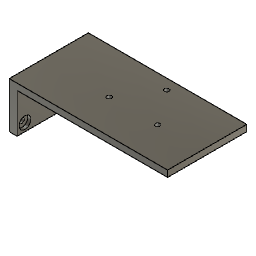
Boat_final_design v3 (Autodesk Fusion 360 archive; units mm, degrees)
design "Plat_servo_cover"
Autodesk Fusion 360 part; units mm, degrees
(part 1 of 7)
sketch "Sketch1" plane through (0, 0, 0) normal (0, 0, 1) x (1, 0, 0)
  line L0 (50, 25) -> (-50, 25)
  line L1 (-50, 25) -> (-50, -25)
  line L2 (-50, -25) -> (50, -25)
  line L3 (50, -25) -> (50, 25)
  line L4 (50, 25) -> (-50, -25) construction
  line L5 (-50, 25) -> (50, -25) construction
  line L6 (-50, 25) -> (-45, 25)
  line L7 (-45, 25) -> (-45, -24.9653)
  line L8 (-45, -24.9653) -> (-50, -24.9653)
  line L9 (-50, -24.9653) -> (-50, 25)
  dimension "d1" = 100
  dimension "d2" = 50
  dimension "d5" = 5
  constraint horizontal L0
  constraint perpendicular L0 L1
  constraint parallel L0 L2
  constraint parallel L1 L3
  constraint coincident L4 origin
  constraint coincident L5 origin
  constraint horizontal L6
  constraint vertical L7
  constraint horizontal L8
  constraint vertical L9
  measures "d1" distance of L1.end L2.end
  measures "d2" distance of L0.end L1.end
  measures "d5" distance of L0.end L6.end
extrude "Extrude1" add sketch "Sketch1" along normal blind 4 makes body 1
extrude "Extrude2" add sketch "Sketch1" against normal blind 25 contours L0 L1 L6 L7 L8 L9 bodies 1
sketch "Sketch2" plane through (0, 0, 0) normal (0, 0, 1) x (1, 0, 0)
  circle A0 centre (-33.372, 3.4391) radius 6.25
  circle A1 centre (-33.372, 9.4391) radius 3.25
  line L0 (50, 25) -> (-50, 25)
  line L1 (-50, -25) -> (50, -25)
  line L2 (-50, -24.9653) -> (-50, 25)
  line L3 (-45, -7.5609) -> (-27.5, -7.5609)
  line L4 (-27.5, -7.5609) -> (-27.5, -2.7609)
  line L5 (-27.5, -2.7609) -> (-45, -2.7609)
  line L6 (-45, -2.7609) -> (-45, -7.5609)
  circle A2 centre (-13.372, 3.4391) radius 3.25
  circle A3 centre (6.628, 3.4391) radius 3.25
  line L7 (-44.814, 24.8891) -> (-27.314, 24.8891)
  line L8 (-27.314, 24.8891) -> (-27.314, 20.0891)
  line L9 (-27.314, 20.0891) -> (-44.814, 20.0891)
  line L10 (-44.814, 20.0891) -> (-44.814, 24.8891)
  dimension "d8" = 12.5
  dimension "d9" = 6.5
  dimension "d15" = 6
  dimension "d17" = 16.628
  dimension "d20" = 17.5
  dimension "d21" = 4.8
  dimension "d47" = 6.5
  dimension "d48" = 20
  dimension "d49" = 6.5
  dimension "d50" = 20
  dimension "d54" = 11
  dimension "d55" = 17.5
  dimension "d56" = 4.8
  dimension "d57" = 32.45
  constraint vertical A0.centre A1.centre
  constraint horizontal L3
  constraint vertical L4
  constraint horizontal L5
  constraint vertical L6
  constraint horizontal A0.centre A2.centre
  constraint horizontal A2.centre A3.centre
  constraint horizontal L7
  constraint vertical L8
  constraint horizontal L9
  constraint vertical L10
  measures "d8" diameter of A0
  measures "d9" diameter of A1
  measures "d15" distance of A0.centre A1.centre
  measures "d17" distance of A0.centre L2
  measures "d20" distance of L3.start L3.end
  measures "d21" distance of L3.start L5.end
  measures "d47" diameter of A2
  measures "d48" horizontal distance of A0.centre A2.centre
  measures "d49" diameter of A3
  measures "d50" horizontal distance of A2.centre A3.centre
  measures "d54" distance of A0.centre L3
  measures "d55" distance of L7.start L7.end
  measures "d56" distance of L7.start L9.end
  measures "d57" distance of L3 L7
sketch "Sketch5" plane through (-45, 0, 0) normal (1, 0, 0) x (0, 1, 0)
  line L0 (-24.9653, 0) -> (-24.9653, -25)
  line L1 (-24.9653, -25) -> (25, -25)
  line L2 (25, -25) -> (25, 0)
  line L3 (25, 0) -> (-24.9653, 0)
  circle A0 centre (20, -20) radius 1.5
  circle A1 centre (-20, -20) radius 1.5
  circle A2 centre (20, -20) radius 3.75
  circle A3 centre (-20, -20) radius 3.75
  line L4 (-8, -9) -> (25, -9)
  line L5 (25, -9) -> (25, -16)
  line L6 (25, -16) -> (-8, -16)
  line L7 (-8, -16) -> (-8, -9)
  dimension "d37" = 3
  dimension "d38" = 3
  dimension "d39" = 5
  dimension "d40" = 40
  dimension "d43" = 7.5
  dimension "d44" = 7.5
  constraint horizontal A0.centre A1.centre
  constraint concentric A0 A2
  constraint concentric A1 A3
  constraint horizontal L4
  constraint vertical L5
  constraint horizontal L6
  constraint vertical L7
  constraint coincident L2 L4.end
  measures "d37" diameter of A0
  measures "d38" diameter of A1
  measures "d39" distance of L1 A0.centre
  measures "d40" distance of A0.centre A1.centre
  measures "d43" diameter of A2
  measures "d44" diameter of A3
extrude "Extrude7" cut sketch "Sketch5" against normal blind 19 contours A0 | A1 bodies 1
extrude "Extrude8" cut sketch "Sketch5" against normal blind 2 contours A2 | A3 bodies 1
sketch "Sketch6" plane through (0, 0, 4) normal (0, 0, 1) x (-1, 0, 0)
  line L0 (50, -25) -> (50, 25)
  line L1 (50, 25) -> (-50, 25)
  line L2 (-50, 25) -> (-50, -25)
  line L3 (-50, -25) -> (50, -25)
  circle A0 centre (8.372, -3.4391) radius 6
  circle A1 centre (-22.128, -3.4391) radius 6
  circle A2 centre (-22.128, -3.4391) radius 1.5
  line L4 (-50, 12.8409) -> (-13.2169, 12.8409) construction
  line L5 (-50, 16.0661) -> (-11, 16.0661) construction
  line L6 (-13.2169, 12.8409) -> (1.2489, 12.8409)
  line L7 (1.2489, 12.8409) -> (1.2489, 24)
  line L8 (1.2489, 24) -> (-13.2169, 24)
  line L9 (-13.2169, 24) -> (-13.2169, 12.8409)
  line L10 (-5.984, 12.8409) -> (-5.984, 24) construction
  line L11 (1.2489, 18.4205) -> (-13.2169, 18.4205) construction
  circle A3 centre (8.372, -3.4391) radius 1.5
  circle A4 centre (-5.984, 18.4205) radius 1.5
  dimension "d80" = 12
  dimension "d93" = 12
  dimension "d94" = 3
  dimension "d98" = 30.5
  dimension "d129" = 1
  dimension "d131" = 3
  dimension "d193" = 3
  constraint concentric A1 A2
  constraint coincident L2 L4.start
  constraint perpendicular L2 L4
  constraint horizontal L5
  constraint coincident L2 L5.start
  constraint horizontal L6
  constraint vertical L7
  constraint horizontal L8
  constraint vertical L9
  constraint midpoint L6 L10.start
  constraint midpoint L8 L10.end
  constraint midpoint L7 L11.start
  constraint midpoint L9 L11.end
  constraint concentric A0 A3
  constraint horizontal A0.centre A1.centre
  constraint midpoint L10 A4.centre
  measures "d80" diameter of A0
  measures "d93" diameter of A1
  measures "d94" diameter of A2
  measures "d98" distance of A0.centre A1.centre
  measures "d129" distance of L1 L8
  measures "d131" diameter of A3
  measures "d193" diameter of A4
extrude "Extrude23" cut sketch "Sketch6" against normal blind 13 contours A2 | A3 | A4 bodies 1
mirror "Mirror1" about plane through (-50, -25, 0) normal (0, -1, 0) of bodies 1 makes body 2
move_body "Move1" bodies 1 to x (1, 0, 0) y (0, 1, 0) z (0, 0, 1) at (0, 35, 0)
hidden bodies 1

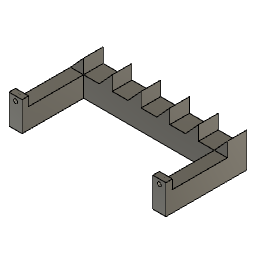
design "Wall_reverse"
Autodesk Fusion 360 part; units mm, degrees
sketch "Sketch1" plane through (0, 0, 0) normal (0, 0, 1) x (1, 0, 0)
  line L0 (30, -7.5) -> (-30, -7.5)
  line L1 (-30, -7.5) -> (-30, 7.5)
  line L2 (-30, 7.5) -> (30, 7.5)
  line L3 (30, 7.5) -> (30, -7.5)
  line L4 (30, -7.5) -> (-30, 7.5) construction
  line L5 (-30, -7.5) -> (30, 7.5) construction
  dimension "d1" = 60
  dimension "d2" = 15
  constraint horizontal L0
  constraint perpendicular L0 L1
  constraint parallel L0 L2
  constraint parallel L1 L3
  constraint coincident L4 origin
  constraint coincident L5 origin
  measures "d1" distance of L1.end L2.end
  measures "d2" distance of L0.end L1.end
extrude "Extrude1" add sketch "Sketch1" along normal blind 15.5 makes body 1
sketch "Sketch2" plane through (0, 0, 15.5) normal (0, 0, 1) x (-1, 0, 0)
  line L0 (-30, -7.5) -> (30, -7.5)
  line L1 (30, -7.5) -> (30, 7.5)
  line L2 (30, 7.5) -> (-30, 7.5)
  line L3 (-30, 7.5) -> (-30, -7.5)
  line L4 (-30, -7.5) -> (-15, -7.5)
  line L5 (-15, -7.5) -> (-15, 12.5)
  line L6 (-15, 12.5) -> (-30, 12.5)
  line L7 (-30, 12.5) -> (-30, -7.5)
  dimension "d5" = 15
  dimension "d6" = 20
  constraint horizontal L4
  constraint vertical L5
  constraint horizontal L6
  constraint vertical L7
  constraint coincident L0.start L3.end
  measures "d5" distance of L0.start L4.end
  measures "d6" distance of L0.start L6.end
sketch "Sketch3" plane through (0, -7.5, 0) normal (0, -1, 0) x (1, 0, 0)
  line L0 (-30, 0) -> (30, 0)
  line L1 (30, 0) -> (30, 15.5)
  line L2 (30, 15.5) -> (-30, 15.5)
  line L3 (-30, 15.5) -> (-30, 0)
  line L4 (20, 15.5) -> (30, 15.5)
  line L5 (30, 15.5) -> (30, 0)
  line L6 (30, 0) -> (20, 0)
  line L7 (20, 0) -> (20, 15.5)
  constraint horizontal L4
  constraint vertical L5
  constraint horizontal L6
  constraint vertical L7
  constraint coincident L0.end L1.start
  constraint coincident L1.end L2.start
extrude "Extrude3" add sketch "Sketch3" along normal blind 47 contours L0 L1 L2 L4 L5 L6 L7 bodies 1
sketch "Sketch4" plane through (0, 0, 15.5) normal (0, 0, 1) x (-1, 0, 0)
  line L0 (-30, 54.5) -> (-30, -7.5)
  line L1 (-20, 7.5) -> (-20, 54.5)
  line L2 (-20, 54.5) -> (-30, 54.5)
  line L3 (-20, 54.5) -> (-61.6412, 54.5)
  line L4 (-61.6412, 54.5) -> (-61.6412, 49.5)
  line L5 (-61.6412, 49.5) -> (-20, 49.5)
  line L6 (-20, 49.5) -> (-20, 54.5)
  line L7 (-30, -7.5) -> (30, -7.5)
  line L8 (30, -7.5) -> (30, 7.5)
  line L9 (30, 7.5) -> (-20, 7.5)
  dimension "d11" = 5
  constraint horizontal L3
  constraint vertical L4
  constraint horizontal L5
  constraint vertical L6
  constraint coincident L1.end L2.start
  measures "d11" distance of L1.end L5.end
extrude "Extrude4" add sketch "Sketch4" along normal blind 7 contours L0 L1 L2 L3 L5 L6 bodies 1
mirror "Mirror1" about plane through (-30, -7.5, 0) normal (-1, 0, 0) of bodies 1 merged
sketch "Sketch5" plane through (0, -49.5, 0) normal (0, 1, 0) x (-1, 0, 0)
  line L0 (80, 15.5) -> (90, 15.5)
  line L1 (90, 15.5) -> (90, 22.5)
  line L2 (90, 22.5) -> (80, 22.5)
  line L3 (80, 22.5) -> (80, 15.5)
  circle A0 centre (-25, 19) radius 3
  circle A1 centre (-25, 19) radius 1.5
  circle A2 centre (85, 19) radius 3
  circle A3 centre (85, 19) radius 1.5
  line L4 (-20, 22.5) -> (-30, 22.5)
  line L5 (-20, 15.5) -> (-20, 22.5)
  dimension "d16" = 6
  dimension "d17" = 3
  dimension "d18" = 6
  dimension "d19" = 3
  dimension "d24" = 3.5
  dimension "d25" = 3.5
  dimension "d40" = 5
  dimension "d41" = 5
  constraint concentric A0 A1
  constraint concentric A2 A3
  measures "d16" diameter of A0
  measures "d17" diameter of A1
  measures "d18" diameter of A2
  measures "d19" diameter of A3
  measures "d24" distance of A0.centre L4
  measures "d25" distance of L2 A2.centre
  measures "d40" distance of A0.centre L5
  measures "d41" distance of L1 A2.centre
extrude "Extrude5" cut sketch "Sketch5" against normal blind 15 contours A1 | A3 bodies 1
extrude "Extrude6" cut sketch "Sketch5" against normal blind 2 contours A0 | A2 bodies 1
sketch "Sketch6" plane through (0, 0, 15.5) normal (0, 0, 1) x (-1, 0, 0)
  line L0 (-20, 49.5) -> (-30, 49.5)
  line L1 (-30, 49.5) -> (-30, -7.5)
  line L2 (-30, -7.5) -> (90, -7.5)
  line L3 (90, -7.5) -> (90, 49.5)
  line L4 (90, 49.5) -> (80, 49.5)
  line L5 (80, 49.5) -> (80, 7.5)
  line L6 (80, 7.5) -> (-20, 7.5)
  line L7 (-20, 7.5) -> (-20, 49.5)
  line L8 (-30, -7.5) -> (-20, -7.5)
  line L9 (-20, -7.5) -> (-20, 7.5)
  line L10 (-20, 7.5) -> (-30, 7.5)
  line L11 (-30, 7.5) -> (-30, -7.5)
  constraint horizontal L8
  constraint vertical L9
  constraint horizontal L10
  constraint vertical L11
  constraint coincident L1.end L2.start
  constraint coincident L6.end L7.start
extrude "Extrude7" add sketch "Sketch6" along normal blind 11 contours L1 L2 L8 L9 L10 L11 bodies 1
sketch "Sketch7" plane through (0, -7.5, 0) normal (0, -1, 0) x (1, 0, 0)
  line L0 (20, 15.5) -> (30, 15.5)
  line L1 (30, 15.5) -> (30, 26.5)
  line L2 (30, 26.5) -> (20, 26.5)
  line L3 (20, 26.5) -> (20, 15.5)
  line L4 (20, 26.5) -> (30, 15.5)
  constraint coincident L2.end L3.start
  constraint coincident L0.end L1.start
extrude "Extrude9" cut sketch "Sketch7" against normal through all contours L1 L2 L4 bodies 1
pattern_linear "R-Pattern2" count 6 spacing 22 along (-1, 0, 0) of "Extrude7", "Extrude9"
mirror "Mirror2" about plane through (0, 0, 0) normal (1, 0, 0) of bodies 1 makes body 2
move_body "Move1" bodies 2 to x (1, 0, 0) y (0, 1, 0) z (0, 0, 1) at (-55, 95, 0)
hidden bodies 1

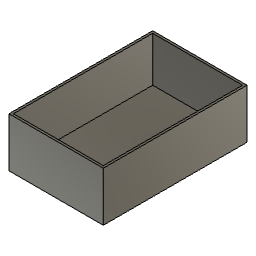
design "ikea box hull"
Autodesk Fusion 360 part; units mm, degrees
sketch "Sketch1" plane through (0, 0, 0) normal (0, 0, 1) x (1, 0, 0)
  line L0 (105, 160) -> (-105, 160)
  line L1 (-105, 160) -> (-105, -160)
  line L2 (-105, -160) -> (105, -160)
  line L3 (105, -160) -> (105, 160)
  line L4 (105, 160) -> (-105, -160) construction
  line L5 (-105, 160) -> (105, -160) construction
  dimension "d1" = 210
  dimension "d2" = 320
  constraint horizontal L0
  constraint perpendicular L0 L1
  constraint parallel L0 L2
  constraint parallel L1 L3
  constraint coincident L4 origin
  constraint coincident L5 origin
  measures "d1" distance of L1.end L2.end
  measures "d2" distance of L0.end L1.end
extrude "Extrude1" add sketch "Sketch1" along normal blind 110
sketch "Sketch2" plane through (0, 0, 110) normal (0, 0, 1) x (-1, 0, 0)
  line L0 (-105, 160) -> (-105, -160)
  line L1 (-105, -160) -> (105, -160)
  line L2 (105, -160) -> (105, 160)
  line L3 (105, 160) -> (-105, 160)
  line L4 (-100, -155) -> (100, -155)
  line L5 (100, -155) -> (100, 155)
  line L6 (100, 155) -> (-100, 155)
  line L7 (-100, 155) -> (-100, -155)
  line L8 (-100, -155) -> (100, 155) construction
  line L9 (100, -155) -> (-100, 155) construction
  dimension "d5" = 200
  dimension "d6" = 310
  constraint horizontal L4
  constraint perpendicular L4 L5
  constraint parallel L4 L6
  constraint parallel L5 L7
  constraint coincident L8 origin
  constraint coincident L9 origin
  measures "d5" distance of L5.end L6.end
  measures "d6" distance of L4.end L5.end
extrude "Extrude2" cut sketch "Sketch2" against normal blind 100 contours L4 L5 L6 L7

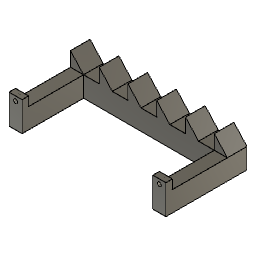
design "Wall"
Autodesk Fusion 360 part; units mm, degrees
sketch "Sketch1" plane through (0, 0, 0) normal (0, 0, 1) x (1, 0, 0)
  line L0 (30, -7.5) -> (-30, -7.5)
  line L1 (-30, -7.5) -> (-30, 7.5)
  line L2 (-30, 7.5) -> (30, 7.5)
  line L3 (30, 7.5) -> (30, -7.5)
  line L4 (30, -7.5) -> (-30, 7.5) construction
  line L5 (-30, -7.5) -> (30, 7.5) construction
  dimension "d1" = 60
  dimension "d2" = 15
  constraint horizontal L0
  constraint perpendicular L0 L1
  constraint parallel L0 L2
  constraint parallel L1 L3
  constraint coincident L4 origin
  constraint coincident L5 origin
  measures "d1" distance of L1.end L2.end
  measures "d2" distance of L0.end L1.end
extrude "Extrude1" add sketch "Sketch1" along normal blind 15.5
sketch "Sketch2" plane through (0, 0, 15.5) normal (0, 0, 1) x (-1, 0, 0)
  line L0 (-30, -7.5) -> (30, -7.5)
  line L1 (30, -7.5) -> (30, 7.5)
  line L2 (30, 7.5) -> (-30, 7.5)
  line L3 (-30, 7.5) -> (-30, -7.5)
  line L4 (-30, -7.5) -> (-15, -7.5)
  line L5 (-15, -7.5) -> (-15, 12.5)
  line L6 (-15, 12.5) -> (-30, 12.5)
  line L7 (-30, 12.5) -> (-30, -7.5)
  dimension "d5" = 15
  dimension "d6" = 20
  constraint horizontal L4
  constraint vertical L5
  constraint horizontal L6
  constraint vertical L7
  constraint coincident L0.start L3.end
  measures "d5" distance of L0.start L4.end
  measures "d6" distance of L0.start L6.end
sketch "Sketch3" plane through (0, -7.5, 0) normal (0, -1, 0) x (1, 0, 0)
  line L0 (-30, 0) -> (30, 0)
  line L1 (30, 0) -> (30, 15.5)
  line L2 (30, 15.5) -> (-30, 15.5)
  line L3 (-30, 15.5) -> (-30, 0)
  line L4 (20, 15.5) -> (30, 15.5)
  line L5 (30, 15.5) -> (30, 0)
  line L6 (30, 0) -> (20, 0)
  line L7 (20, 0) -> (20, 15.5)
  constraint horizontal L4
  constraint vertical L5
  constraint horizontal L6
  constraint vertical L7
  constraint coincident L0.end L1.start
  constraint coincident L1.end L2.start
extrude "Extrude3" add sketch "Sketch3" along normal blind 47 contours L0 L1 L2 L4 L5 L6 L7
sketch "Sketch4" plane through (0, 0, 15.5) normal (0, 0, 1) x (-1, 0, 0)
  line L0 (-30, 54.5) -> (-30, -7.5)
  line L1 (-20, 7.5) -> (-20, 54.5)
  line L2 (-20, 54.5) -> (-30, 54.5)
  line L3 (-20, 54.5) -> (-61.6412, 54.5)
  line L4 (-61.6412, 54.5) -> (-61.6412, 49.5)
  line L5 (-61.6412, 49.5) -> (-20, 49.5)
  line L6 (-20, 49.5) -> (-20, 54.5)
  line L7 (-30, -7.5) -> (30, -7.5)
  line L8 (30, -7.5) -> (30, 7.5)
  line L9 (30, 7.5) -> (-20, 7.5)
  dimension "d11" = 5
  constraint horizontal L3
  constraint vertical L4
  constraint horizontal L5
  constraint vertical L6
  constraint coincident L1.end L2.start
  measures "d11" distance of L1.end L5.end
extrude "Extrude4" add sketch "Sketch4" along normal blind 7 contours L0 L1 L2 L3 L5 L6
mirror "Mirror1" about plane through (-30, -7.5, 0) normal (-1, 0, 0) of bodies 1 merged
sketch "Sketch5" plane through (0, -49.5, 0) normal (0, 1, 0) x (-1, 0, 0)
  line L0 (80, 15.5) -> (90, 15.5)
  line L1 (90, 15.5) -> (90, 22.5)
  line L2 (90, 22.5) -> (80, 22.5)
  line L3 (80, 22.5) -> (80, 15.5)
  circle A0 centre (-25, 19) radius 3
  circle A1 centre (-25, 19) radius 1.5
  circle A2 centre (85, 19) radius 3
  circle A3 centre (85, 19) radius 1.5
  line L4 (-20, 22.5) -> (-30, 22.5)
  line L5 (-20, 15.5) -> (-20, 22.5)
  dimension "d16" = 6
  dimension "d17" = 3
  dimension "d18" = 6
  dimension "d19" = 3
  dimension "d24" = 3.5
  dimension "d25" = 3.5
  dimension "d40" = 5
  dimension "d41" = 5
  constraint concentric A0 A1
  constraint concentric A2 A3
  measures "d16" diameter of A0
  measures "d17" diameter of A1
  measures "d18" diameter of A2
  measures "d19" diameter of A3
  measures "d24" distance of A0.centre L4
  measures "d25" distance of L2 A2.centre
  measures "d40" distance of A0.centre L5
  measures "d41" distance of L1 A2.centre
extrude "Extrude5" cut sketch "Sketch5" against normal blind 15 contours A1 | A3
extrude "Extrude6" cut sketch "Sketch5" against normal blind 2 contours A0 | A2
sketch "Sketch6" plane through (0, 0, 15.5) normal (0, 0, 1) x (-1, 0, 0)
  line L0 (-20, 49.5) -> (-30, 49.5)
  line L1 (-30, 49.5) -> (-30, -7.5)
  line L2 (-30, -7.5) -> (90, -7.5)
  line L3 (90, -7.5) -> (90, 49.5)
  line L4 (90, 49.5) -> (80, 49.5)
  line L5 (80, 49.5) -> (80, 7.5)
  line L6 (80, 7.5) -> (-20, 7.5)
  line L7 (-20, 7.5) -> (-20, 49.5)
  line L8 (-30, -7.5) -> (-20, -7.5)
  line L9 (-20, -7.5) -> (-20, 7.5)
  line L10 (-20, 7.5) -> (-30, 7.5)
  line L11 (-30, 7.5) -> (-30, -7.5)
  constraint horizontal L8
  constraint vertical L9
  constraint horizontal L10
  constraint vertical L11
  constraint coincident L1.end L2.start
  constraint coincident L6.end L7.start
extrude "Extrude7" add sketch "Sketch6" along normal blind 11 contours L1 L2 L8 L9 L10 L11
sketch "Sketch7" plane through (0, -7.5, 0) normal (0, -1, 0) x (1, 0, 0)
  line L0 (20, 15.5) -> (30, 15.5)
  line L1 (30, 15.5) -> (30, 26.5)
  line L2 (30, 26.5) -> (20, 26.5)
  line L3 (20, 26.5) -> (20, 15.5)
  line L4 (20, 26.5) -> (30, 15.5)
  constraint coincident L2.end L3.start
  constraint coincident L0.end L1.start
extrude "Extrude9" cut sketch "Sketch7" against normal through all contours L1 L2 L4
pattern_linear "R-Pattern2" count 6 spacing 22 along (-1, 0, 0) of "Extrude7", "Extrude9"

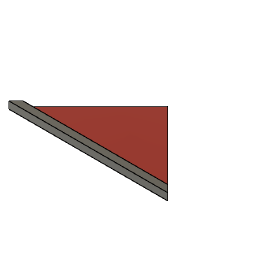
design "New_sqaure"
Autodesk Fusion 360 part; units mm, degrees
sketch "Sketch1" plane through (0, 0, 0) normal (0, 0, 1) x (1, 0, 0)
  line L0 (0, 0) -> (0, 112)
  line L1 (0, 0) -> (112, 0)
  line L2 (0, 112) -> (112, 0)
  line L3 (0, 112) -> (-112, 0)
  line L4 (0, 0) -> (-112, 0)
  dimension "d3" = 112
  dimension "d4" = 112
  dimension "d5" = 158.3919
  constraint coincident L0.start L1.start
  constraint vertical L0
  constraint perpendicular L0 L1
  constraint symmetric L2.start L0 L3.start
  constraint symmetric L0 L1.start L4.start
  constraint symmetric L0 L1.end L3.end
  measures "d3" distance of L0.start L0.end
  measures "d4" distance of L0.start L1.end
  measures "d5" distance of L0.end L1.end
extrude "Extrude1" add sketch "Sketch1" along normal blind 3
sketch "Sketch2" plane through (0, 0, 0) normal (0, 0, -1) x (1, 0, 0)
  line L0 (-112, 0) -> (0, -112)
  line L1 (0, -112) -> (112, 0)
  line L2 (112, 0) -> (-112, 0)
  line L3 (0, 0) -> (0, -10) construction
  line L4 (0, -10) -> (115, -10)
  line L5 (115, -10) -> (-102, -10)
  dimension "d8" = 10
  constraint coincident L3.start origin
  constraint perpendicular L2 L3
  constraint perpendicular L3 L4
  constraint coincident L0 L5.end
  constraint perpendicular L3 L5
  measures "d8" distance of L3.start L3.end
sketch "Sketch3" plane through (0, 0, 3) normal (0, 0, 1) x (-1, 0, 0)
  line L0 (0, -112) -> (112, 0)
  line L1 (112, 0) -> (-112, 0)
  line L2 (-112, 0) -> (0, -112)
  line L3 (0, 0) -> (0, -10) construction
  line L4 (0, -10) -> (115, -10)
  line L5 (115, -10) -> (-102, -10)
  dimension "d11" = 10
  constraint coincident L3.start origin
  constraint perpendicular L1 L3
  constraint perpendicular L3 L4
  constraint coincident L2 L5.end
  constraint perpendicular L3 L5
  measures "d11" distance of L3.start L3.end
extrude "Extrude3" add sketch "Sketch3" along normal blind 7 contours L0 L1 L2 L4 L5
sketch "Sketch4" plane through (0, 0, 0) normal (0, -1, 0) x (1, 0, 0)
  line L0 (112, 0) -> (112, 10)
  line L1 (112, 10) -> (-112, 10)
  line L2 (-112, 10) -> (-112, 0)
  line L3 (0, 0) -> (-112, 0)
  line L4 (0, 0) -> (112, 0)
  line L5 (-112, 0) -> (112, 0)
  constraint coincident L3.start L4.start
  constraint coincident L2 L3.end
  constraint perpendicular L2 L3
  constraint coincident L0 L4.end
  constraint perpendicular L0 L4
extrude "Extrude4" [suppressed]
equation "Height_lenght = 112 mm"
equation "Sqaure_lenght = sqrt(2) * Height_lenght"
equation "d3 = Height_lenght"
equation "d4 = Height_lenght"
equation "d5 = Sqaure_lenght"

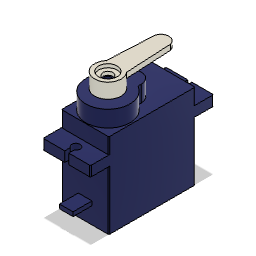
design "SG90 9g servo"
Autodesk Fusion 360 part; units mm, degrees
sketch "Body" plane through (0, 0, 0) normal (0, 1, 0) x (1, 0, 0) in component "servo"
  line L0 (6.25, -11.375) -> (-6.25, -11.375)
  line L1 (-6.25, -11.375) -> (-6.25, 11.375)
  line L2 (-6.25, 11.375) -> (6.25, 11.375)
  line L3 (6.25, 11.375) -> (6.25, -11.375)
  line L4 (6.25, -11.375) -> (-6.25, 11.375) construction
  line L5 (-6.25, -11.375) -> (6.25, 11.375) construction
  dimension "d6" = 12.5
  dimension "d7" = 22.75
  dimension "d52" = 0
  dimension "d53" = 0
  dimension "d54" = 0
  dimension "d55" = 0
  constraint perpendicular L0 L1
  constraint parallel L0 L2
  constraint parallel L1 L3
  constraint horizontal L0
  constraint coincident L4 origin
  constraint coincident L5 origin
  measures "d6" distance of L1.end L2.end
  measures "d7" distance of L0.end L1.end
extrude "Extrude1" add sketch "Body" along normal blind 22.35 makes body 1 in component "servo"
sketch "Tab" plane through (0, 0, 11.375) normal (0, 0, 1) x (1, 0, 0) in component "servo"
  line L0 (-6.25, 0) -> (6.25, 0)
  line L1 (6.25, 0) -> (6.25, 22.35)
  line L2 (6.25, 22.35) -> (-6.25, 22.35)
  line L3 (-6.25, 22.35) -> (-6.25, 0)
  line L4 (-6.25, 18.2) -> (6.25, 18.2)
  line L5 (6.25, 18.2) -> (6.25, 15.55)
  line L6 (6.25, 15.55) -> (-6.25, 15.55)
  line L7 (-6.25, 15.55) -> (-6.25, 18.2)
  dimension "d10" = 4.15
  dimension "d11" = 2.65
  constraint horizontal L4
  constraint vertical L5
  constraint horizontal L6
  constraint vertical L7
  constraint coincident L1 L5.end
  constraint coincident L3 L4.start
  measures "d10" distance of L1.end L4.end
  measures "d11" distance of L4.end L5.end
extrude "Extrude2" add sketch "Tab" along normal blind 4.85 contours L1 L3 L4 L5 L6 L7 bodies 1 in component "servo"
hole "Hole1" at (0, 18.2, 13.8) direction (0, -1, 0) diameter 2.2 end through all bodies 1 in component "servo"
fillet "Fillet1" radius 0.25 2 edges at (6.25, 16.875, 16.225) (-6.25, 16.875, 16.225) on bodies 1 in component "servo"
sketch "Notch" plane through (0, 0, 16.225) normal (0, 0, 1) x (1, 0, 0) in component "servo"
  line L0 (-6, 18.2) -> (-6, 15.55)
  line L1 (-6, 15.55) -> (6, 15.55)
  line L2 (6, 15.55) -> (6, 18.2)
  line L3 (6, 18.2) -> (-6, 18.2)
  line L4 (-0.525, 18.2) -> (0.525, 18.2)
  line L5 (0.525, 18.2) -> (0.525, 15.55)
  line L6 (0.525, 15.55) -> (-0.525, 15.55)
  line L7 (-0.525, 15.55) -> (-0.525, 18.2)
  dimension "d20" = 1.05
  constraint collinear L3 L4
  constraint collinear L1 L6
  constraint parallel L5 L7
  measures "d20" distance of L4.start L4.end
extrude "Extrude3" cut sketch "Notch" along normal up to surface contours L1 L3 L4 L5 L6 L7 end surface at (0.0548, 17.3167, 14.8986) on bodies 1 bodies 1 in component "servo"
mirror "Mirror1" about plane through (0, 0, 0) normal (0, 0, 1) of "Extrude2", "Hole1", "Fillet1", "Extrude3" in component "servo"
sketch "Bump" plane through (0, 22.35, 0) normal (0, 1, 0) x (-1, 0, 0) in component "servo"
  line L0 (-6.25, -11.375) -> (6.25, -11.375)
  line L1 (6.25, -11.375) -> (6.25, 11.375)
  line L2 (6.25, 11.375) -> (-6.25, 11.375)
  line L3 (-6.25, 11.375) -> (-6.25, -11.375)
  line L4 (-2.8, -0.625) -> (-2.8, 0.2671)
  line L5 (2.8, 0.2671) -> (2.8, -0.625)
  arc A0 (-2.8, -0.625) -> (2.8, -0.625) centre (0, -0.625) ccw
  arc A1 (2.8, 0.2671) -> (-2.8, 0.2671) centre (0, 5.375) ccw
  dimension "d23" = 11.65
  dimension "d24" = 6
  dimension "d25" = 5.6
  dimension "d26" = 6
  dimension "d27" = 6.25
  dimension "d28" = 6.25
  constraint tangent L4 A0
  constraint vertical L4
  constraint tangent L5 A0
  measures "d23" diameter of A1
  measures "d24" distance of L2 A1.centre
  measures "d25" diameter of A0
  measures "d26" distance of A1.centre A0.centre
  measures "d27" distance of L3 A1.centre
  measures "d28" distance of L3 A0.centre
extrude "Extrude4" add sketch "Bump" along normal blind 4.3 contours L4 L5 A0 A1 bodies 1 in component "servo"
fillet "Fillet2" radius 0.25 8 edges at (6.25, 7.775, 11.375) (6.25, 20.275, 11.375) (-6.25, 20.275, 11.375) (-6.25, 7.775, 11.375) (6.25, 7.775, -11.375) (6.25, 20.275, -11.375) (-6.25, 20.275, -11.375) (-6.25, 7.775, -11.375) on bodies 1 in component "servo"
hole "Hole2" at (0, 26.65, 5.375) direction (0, -1, 0) diameter 4.92 depth 15 tip angle 180 bodies 1 in component "servo"
sketch "Wire" plane through (0, 0, 11.375) normal (0, 0, 1) x (1, 0, 0) in component "servo"
  line L0 (-6, 15.55) -> (-6, 0)
  line L1 (-6, 0) -> (6, 0)
  line L2 (6, 0) -> (6, 15.55)
  line L3 (6, 15.55) -> (-6, 15.55)
  line L4 (-1.8, 5.5) -> (1.8, 5.5)
  line L5 (1.8, 5.5) -> (1.8, 4.4)
  line L6 (1.8, 4.4) -> (-1.8, 4.4)
  line L7 (-1.8, 4.4) -> (-1.8, 5.5)
  dimension "d32" = 1.1
  dimension "d33" = 3.6
  dimension "d34" = 5.5
  constraint horizontal L4
  constraint vertical L5
  constraint horizontal L6
  constraint vertical L7
  measures "d32" distance of L4.start L6.end
  measures "d33" distance of L4.start L4.end
  measures "d34" distance of L1 L4.end
extrude "Extrude5" add sketch "Wire" along normal blind 5 contours L4 L5 L6 L7 bodies 1 in component "servo"
cylinder "CylinderPrimitive1" add diameter 4.92 height 2.72 placed x (1, 0, 0) y (0, 0, -1) z (0, 1, 0) at (0, 26.65, 5.375) separate body makes body 2 in component "splined-drive"
extrude "Extrude1'" add 1 faces at (-0.4548, 26.65, 5.9711) along direction (0, -1, 0) blind 15 on bodies 2 bodies 2 in component "splined-drive"
hole "Hole1'" at (0, 29.37, 5.375) direction (0, -1, 0) diameter 1.95 depth 5 tip angle 180 bodies 2 in component "splined-drive"
chamfer "Chamfer1" distance 0.25 angle 45 1 edges at (-2.2935, 29.37, 6.2646) on bodies 2 in component "splined-drive"
sketch "Sketch1" plane through (0, 29.37, 0) normal (0, 1, 0) x (-1, 0, 0) in component "horn"
  circle A0 centre (0, 5.375) radius 3.5
  circle A1 centre (0, 5.375) radius 2.46
  circle A2 centre (0, 5.375) radius 1.31
  dimension "d102" = 0
  dimension "d103" = 0
  dimension "d104" = 0
  dimension "d105" = 0
extrude "Extrude3'" add sketch "Sketch1" against normal blind 2.08 separate body contours A0 makes body 3 in component "horn"
extrude "Extrude6" add 1 faces at (-3.1311, 29.37, 5.0789) along direction (0, 1, 0) blind 1.83 on bodies 3 bodies 3 in component "horn"
extrude "Extrude4'" add sketch "Sketch1" along normal blind 0.9 contours A1 bodies 3 in component "horn"
sketch "Sketch4" plane through (0, 31.2, 0) normal (0, 1, 0) x (-1, 0, 0) in component "horn"
  circle A0 centre (0, 5.375) radius 2.46
  circle A1 centre (0, 5.375) radius 3.5
  line L0 (2.67, 3.112) -> (2.04, -9.105)
  line L1 (-2.67, 3.112) -> (-2.04, -9.105)
  arc A2 (-2.04, -9.105) -> (2.04, -9.105) centre (0, -8.6045) ccw
  constraint coincident A1 L0.start
  constraint coincident A1 L1.start
extrude "Extrude7" add sketch "Sketch4" against normal blind 1.41 contours A1 L0 L1 A2 bodies 3 in component "horn"
component "servo" placed x (1, 0, 0) y (0, 1, 0) z (0, 0, 1) at (0, 0, 0)
component "splined-drive" placed x (1, 0, 0) y (0, 1, 0) z (0, 0, 1) at (0, 0, 0)
component "horn" placed x (1, 0, 0) y (0, 1, 0) z (0, 0, 1) at (0, 0, 0)

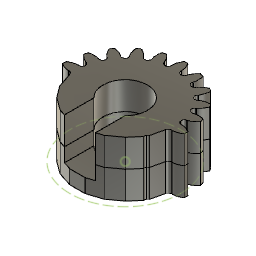
design "Servo_gear"
description: Spur Gear; Module: 1.000000; Num Teeth: 20; Pressure Angle: 20.000000; Backlash: 0.00 mm
Autodesk Fusion 360 part; units mm, degrees
sketch "Sketch1" plane through (0, 0, 0) normal (0, 0, 1) x (1, 0, 0) in component "Spur Gear (20 teeth)"
  circle A0 centre (0, 0) radius 8.7492
  circle A1 centre (0, 0) radius 3.5
extrude "Extrude1" add sketch "Sketch1" along normal blind 5 makes body 1 in component "Spur Gear (20 teeth)"
sketch "Sketch2" plane through (0, 0, 0) normal (0, 0, 1) x (1, 0, 0) in component "Spur Gear (20 teeth)"
  spline S0 degree 5 poles (9.3559, -0.8768) (9.3606, -0.8772) (9.3699, -0.878) (9.3839, -0.8787) (9.4026, -0.879) (9.426, -0.8784) (9.4495, -0.8772) (9.473, -0.8755) (9.4965, -0.8735) (9.52, -0.8714) (9.5435, -0.8691) (9.567, -0.8666) (9.5906, -0.8638) (9.6142, -0.8607) (9.6377, -0.8572) (9.6613, -0.8534) (9.6849, -0.8494) (9.7085, -0.8451) (9.7321, -0.8406) (9.7557, -0.836) (9.7793, -0.8311) (9.8029, -0.8261) (9.8265, -0.8208) (9.8501, -0.8153) (9.8737, -0.8096) (9.8973, -0.8037) (9.9209, -0.7977) (9.9445, -0.7914) (9.968, -0.7849) (9.9916, -0.7783) (10.0152, -0.7715) (10.0388, -0.7645) (10.0623, -0.7574) (10.0859, -0.7501) (10.1095, -0.7426) (10.133, -0.7349) (10.1565, -0.7271) (10.1801, -0.7191) (10.2036, -0.711) (10.2271, -0.7027) (10.2506, -0.6942) (10.2741, -0.6856) (10.2976, -0.6768) (10.321, -0.6679) (10.3445, -0.6588) (10.3679, -0.6496) (10.3913, -0.6402) (10.4148, -0.6307) (10.4382, -0.621) (10.4615, -0.6112) (10.4849, -0.6013) (10.5083, -0.5912) (10.5316, -0.5809) (10.5549, -0.5705) (10.5782, -0.56) (10.6015, -0.5493) (10.6248, -0.5385) (10.6481, -0.5276) (10.6713, -0.5165) (10.6945, -0.5053) (10.7177, -0.4939) (10.7409, -0.4824) (10.7641, -0.4708) (10.7872, -0.4591) (10.8103, -0.4472) (10.8334, -0.4352) (10.8565, -0.423) (10.8796, -0.4107) (10.9026, -0.3983) (10.9256, -0.3858) (10.9486, -0.3731) (10.967, -0.3629) (10.9807, -0.3552) (10.9899, -0.35) (10.9945, -0.3474) knots 0 0 0 0 0 0 0.01428571 0.02857143 0.04285714 0.05714286 0.07142857 0.08571429 0.1 0.11428571 0.12857143 0.14285714 0.15714286 0.17142857 0.18571429 0.2 0.21428571 0.22857143 0.24285714 0.25714286 0.27142857 0.28571429 0.3 0.31428571 0.32857143 0.34285714 0.35714286 0.37142857 0.38571429 0.4 0.41428571 0.42857143 0.44285714 0.45714286 0.47142857 0.48571429 0.5 0.51428571 0.52857143 0.54285714 0.55714286 0.57142857 0.58571429 0.6 0.61428571 0.62857143 0.64285714 0.65714286 0.67142857 0.68571429 0.7 0.71428571 0.72857143 0.74285714 0.75714286 0.77142857 0.78571429 0.8 0.81428571 0.82857143 0.84285714 0.85714286 0.87142857 0.88571429 0.9 0.91428571 0.92857143 0.94285714 0.95714286 0.97142857 0.98571429 1 1 1 1 1 1
  spline S1 degree 5 poles (9.3559, 0.8768) (9.3606, 0.8772) (9.3699, 0.878) (9.3839, 0.8787) (9.4026, 0.879) (9.426, 0.8784) (9.4495, 0.8772) (9.473, 0.8755) (9.4965, 0.8735) (9.52, 0.8714) (9.5435, 0.8691) (9.567, 0.8666) (9.5906, 0.8638) (9.6142, 0.8607) (9.6377, 0.8572) (9.6613, 0.8534) (9.6849, 0.8494) (9.7085, 0.8451) (9.7321, 0.8406) (9.7557, 0.836) (9.7793, 0.8311) (9.8029, 0.8261) (9.8265, 0.8208) (9.8501, 0.8153) (9.8737, 0.8096) (9.8973, 0.8037) (9.9209, 0.7977) (9.9445, 0.7914) (9.968, 0.7849) (9.9916, 0.7783) (10.0152, 0.7715) (10.0388, 0.7645) (10.0623, 0.7574) (10.0859, 0.7501) (10.1095, 0.7426) (10.133, 0.7349) (10.1565, 0.7271) (10.1801, 0.7191) (10.2036, 0.711) (10.2271, 0.7027) (10.2506, 0.6942) (10.2741, 0.6856) (10.2976, 0.6768) (10.321, 0.6679) (10.3445, 0.6588) (10.3679, 0.6496) (10.3913, 0.6402) (10.4148, 0.6307) (10.4382, 0.621) (10.4615, 0.6112) (10.4849, 0.6013) (10.5083, 0.5912) (10.5316, 0.5809) (10.5549, 0.5705) (10.5782, 0.56) (10.6015, 0.5493) (10.6248, 0.5385) (10.6481, 0.5276) (10.6713, 0.5165) (10.6945, 0.5053) (10.7177, 0.4939) (10.7409, 0.4824) (10.7641, 0.4708) (10.7872, 0.4591) (10.8103, 0.4472) (10.8334, 0.4352) (10.8565, 0.423) (10.8796, 0.4107) (10.9026, 0.3983) (10.9256, 0.3858) (10.9486, 0.3731) (10.967, 0.3629) (10.9807, 0.3552) (10.9899, 0.35) (10.9945, 0.3474) knots 0 0 0 0 0 0 0.01428571 0.02857143 0.04285714 0.05714286 0.07142857 0.08571429 0.1 0.11428571 0.12857143 0.14285714 0.15714286 0.17142857 0.18571429 0.2 0.21428571 0.22857143 0.24285714 0.25714286 0.27142857 0.28571429 0.3 0.31428571 0.32857143 0.34285714 0.35714286 0.37142857 0.38571429 0.4 0.41428571 0.42857143 0.44285714 0.45714286 0.47142857 0.48571429 0.5 0.51428571 0.52857143 0.54285714 0.55714286 0.57142857 0.58571429 0.6 0.61428571 0.62857143 0.64285714 0.65714286 0.67142857 0.68571429 0.7 0.71428571 0.72857143 0.74285714 0.75714286 0.77142857 0.78571429 0.8 0.81428571 0.82857143 0.84285714 0.85714286 0.87142857 0.88571429 0.9 0.91428571 0.92857143 0.94285714 0.95714286 0.97142857 0.98571429 1 1 1 1 1 1
  arc A0 (10.9945, -0.3474) -> (10.9945, 0.3474) centre (0, 0) ccw
  line L0 (8.7011, -0.8164) -> (9.3559, -0.8768)
  line L1 (8.7011, 0.8164) -> (9.3559, 0.8768)
  line L2 (8.7011, -0.8164) -> (8.7011, 0.8164)
  point P0 (9.471, -0.8756)
  point P1 (9.5871, -0.8642)
  point P2 (9.7036, -0.846)
  point P3 (9.8206, -0.8221)
  point P4 (9.9379, -0.7931)
  point P5 (10.0553, -0.7595)
  point P6 (10.1729, -0.7215)
  point P7 (10.2906, -0.6794)
  point P8 (10.4082, -0.6333)
  point P9 (10.5258, -0.5834)
  point P10 (10.6433, -0.5298)
  point P11 (10.7606, -0.4725)
  point P12 (10.8777, -0.4117)
  point P13 (9.471, 0.8756)
  point P14 (9.5871, 0.8642)
  point P15 (9.7036, 0.846)
  point P16 (9.8206, 0.8221)
  point P17 (9.9379, 0.7931)
  point P18 (10.0553, 0.7595)
  point P19 (10.1729, 0.7215)
  point P20 (10.2906, 0.6794)
  point P21 (10.4082, 0.6333)
  point P22 (10.5258, 0.5834)
  point P23 (10.6433, 0.5298)
  point P24 (10.7606, 0.4725)
  point P25 (10.8777, 0.4117)
extrude "Extrude2" add sketch "Sketch2" along normal blind 5 bodies 1 in component "Spur Gear (20 teeth)"
fillet "Fillet1" radius 0.59 2 edges at (8.7109, -0.8173, 2.5) (8.7109, 0.8173, 2.5) on bodies 1 in component "Spur Gear (20 teeth)"
pattern_circular "C-Pattern1" count 20 over 360 about axis through (0, 0, 0) along (0, 0, 1) of "Extrude2", "Fillet1" in component "Spur Gear (20 teeth)"
sketch "Sketch3" plane through (0, 0, 0) normal (0, 0, 1) x (1, 0, 0) in component "Spur Gear (20 teeth)"
  circle A0 centre (0, 0) radius 10 construction